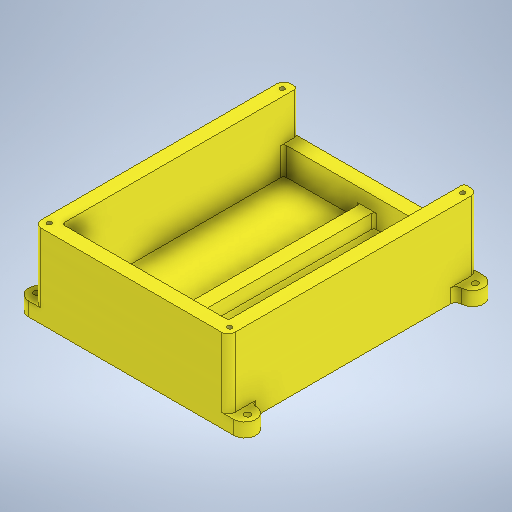
# Autodesk Inventor part: акб корпус
Saved by Autodesk Inventor 2025 (Build 290162000, 162)
## iProperties
Created: 2025-02-25
Part Number: акб корпус
Material: Типовые
Document SubType Name: Modeling
Designer: volko
Density: 1 g/cm^3
Appearance: Канареечный
Author: volko
Autodesk Inventor part; units mm, degrees
ref_plane "YZ Plane" through (0, 0, 0) normal (1, 0, 0) x (0, 1, 0)
ref_plane "XZ Plane" through (0, 0, 0) normal (0, 1, 0) x (-1, 0, 0)
ref_plane "XY Plane" through (0, 0, 0) normal (0, 0, 1) x (1, 0, 0)
sketch "Эскиз1" plane through (0, 0, 0) normal (0, 1, 0) x (-1, 0, 0)
  line L0 (60, 80) -> (-60, 80)
  line L1 (-60, 80) -> (-60, -80)
  line L2 (-60, -80) -> (60, -80)
  line L3 (60, -80) -> (60, 80)
  line L4 (74, 90) -> (-74, 90)
  line L5 (-70, 90) -> (-70, -90)
  line L6 (-74, -90) -> (74, -90)
  line L7 (70, -90) -> (70, 90)
  line L8 (-114.8, 0) -> (114.8, 0) projected
  line L9 (0, -126) -> (0, 126) projected
  line L10 (5, -80) -> (-5, -80)
  line L11 (-5, -80) -> (-5, 80)
  line L12 (-5, 80) -> (5, 80)
  line L13 (5, 80) -> (5, -80)
  arc A0 (-74, 90) -> (-74, 74) centre (-74, 82) ccw
  arc A1 (-70, 70) -> (-74, 74) centre (-74, 70) ccw
  line L14 (-74, 90) -> (-74, 74) construction
  arc A2 (74, 74) -> (74, 90) centre (74, 82) ccw
  arc A3 (74, 74) -> (70, 70) centre (74, 70) ccw
  arc A4 (-74, -74) -> (-74, -90) centre (-74, -82) ccw
  arc A5 (-74, -74) -> (-70, -70) centre (-74, -70) ccw
  arc A6 (74, -90) -> (74, -74) centre (74, -82) ccw
  arc A7 (70, -70) -> (74, -74) centre (74, -70) ccw
  point P0 (0, 0)
  point P1 (5, 80)
  point P2 (-5, -80)
  point P3 (-82, 82)
  dimension "d12" = 160
  dimension "d14" = 55
  dimension "d15" = 10
  dimension "d16" = 10
  dimension "d17" = 10
  dimension "d25" = 8
  dimension "d26" = 12
  constraints: 26 end point, 17 point on circle, 15 symmetric about line, 10 point on line, 8 centre point, 6 parallel, 3 horizontal, 3 perpendicular, 3 tangent, 1 vertical, 11 other
  measures "d12" distance of L2.end L0.start
  measures "d14" distance between parallel lines of L13 L3
  measures "d15" distance between parallel lines of L11 L13
  measures "d16" distance between parallel lines of L5 L1
  measures "d17" distance between parallel lines of L2 L6
  measures "d25" radius of A0
  measures "d26" distance from line of point (-82, 82) L5
extrude "Выдавливание2" add sketch "Эскиз1" along normal blind 10
extrude "Выдавливание5" add sketch "Эскиз1" along normal blind 20 contours L13 L8 L9 L0 | L9 L8 L11 L0 | L13 L2 L9 L8 | L9 L2 L11 L8
extrude "Выдавливание7" add sketch "Эскиз1" along normal blind 60 contours L0 L9 L4 L7 L8 L3 | L8 L7 L6 L9 L2 L3 | L0 L1 L8 L5 L4 L9 | L9 L6 L5 L8 L1 L2
fillet "Сопряжение2" radius 5 4 edges at (70, 35, -90) (70, 35, 90) (-70, 35, -90) (-70, 35, 90)
sketch "Эскиз6" plane through (0, 0, 0) normal (0, 0, 1) x (1, 0, 0)
  line L0 (60, 10) -> (60, 60) projected
  line L1 (-60, 10) -> (-60, 60) projected
  line L2 (60, 60) -> (-60, 60)
  line L3 (-60, 60) -> (-60, 30)
  line L4 (-60, 30) -> (60, 30)
  line L5 (60, 30) -> (60, 60)
  point P0 (0, 0)
  dimension "d30" = 30
  constraints: 8 end point, 2 parallel, 1 horizontal, 1 perpendicular, 1 point on line
  measures "d30" distance between parallel lines of L4 L2
extrude "Выдавливание8" cut sketch "Эскиз6" against normal through all
fillet "Сопряжение3" radius 2 10 edges at (60, 35, 80) (-60, 35, 80) (5, 15, 80) (-5, 15, 80) (5, 15, -80) (60, 20, -80) (-5, 15, -80) (-60, 20, -80) (60, 45, -90) (-60, 45, -90)
sketch "Эскиз7" plane through (0, 10, 0) normal (0, 1, 0) x (1, 0, 0)
  line L0 (-114.8, 0) -> (114.8, 0) projected
  line L1 (0, 126) -> (0, -126) projected
  line L2 (-62, 90) -> (62, 90) projected
  line L3 (-70, 70) -> (-70, 85) projected
  arc A0 (-65, 90) -> (-70, 85) centre (-65, 85) ccw projected
  line L4 (-65, 90) -> (-74, 90) projected
  arc A1 (-74, 90) -> (-74, 74) centre (-74, 82) ccw projected
  arc A2 (-70, 70) -> (-74, 74) centre (-74, 70) ccw projected
  line L5 (-70, 85) -> (-70, -85) projected
  point P0 (0, 0)
  point P1 (-76, 82)
  point P2 (-76, -82)
  point P3 (76, 82)
  point P4 (76, -82)
  dimension "d43" = 164
  dimension "d46" = 152
  dimension "d49" = 8
  dimension "d50" = 6
  constraints: 1 horizontal, 1 vertical, 3 other
  measures "d43" distance of point (-76, 82) point (-76, -82)
  measures "d46" distance of point (-76, 82) point (76, 82)
  measures "d49" distance from line of L2 point (-76, 82)
  measures "d50" distance from line of point (-76, 82) L5
hole "Отверстие1" at (-76, 10, -82) at (76, 10, -82) at (-76, 10, 82) at (76, 10, 82) direction (0, -1, 0) diameter 4.5 end through all
sketch "Эскиз8" plane through (0, 60, 0) normal (0, 1, 0) x (1, 0, 0)
  line L0 (0, 126) -> (0, -126) projected
  line L1 (-114.8, 0) -> (114.8, 0) projected
  line L2 (-60, -78) -> (-60, 88) projected
  line L3 (-65, -90) -> (65, -90) projected
  point P0 (0, 0)
  point P1 (-65, -84)
  point P2 (-65, 84)
  point P3 (65, -84)
  point P4 (65, 84)
  dimension "d60" = 168
  dimension "d63" = 130
  dimension "d66" = 5
  dimension "d67" = 6
  constraints: 1 horizontal, 1 vertical, 3 other
  measures "d60" distance of point (-65, -84) point (-65, 84)
  measures "d63" distance of point (-65, -84) point (65, -84)
  measures "d66" distance from line of point (-65, -84) L2
  measures "d67" distance from line of point (-65, -84) L3
hole "Отверстие2" at (-65, 60, 84) at (65, 60, 84) at (65, 60, -84) at (-65, 60, -84) direction (0, -1, 0) diameter 3.242 depth 11.8 tip angle 118 thread size "M4x0.7" class "6H" standard "ISO Metric profile"
